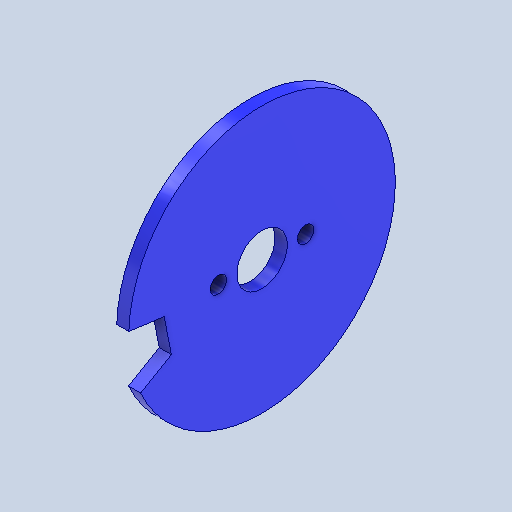
# Autodesk Inventor part: belt_liner_v1_3DP_P_F-1
Saved by Autodesk Inventor 2025.1 (Build 291241000, 241)
## iProperties
Created: 2024-12-16
Part Number: belt_liner_v1_3DP_P_F-1
Material: ABS プラスチック
Document SubType Name: Modeling
Designer: haruy
Density: 1.06 g/cm^3
Appearance: 青 - 壁塗料 - 光沢
Author: haruy
Autodesk Inventor part; units mm, degrees
ref_plane "YZ Plane" through (0, 0, 0) normal (1, 0, 0) x (0, 1, 0)
ref_plane "XZ Plane" through (0, 0, 0) normal (0, 1, 0) x (-1, 0, 0)
ref_plane "XY Plane" through (0, 0, 0) normal (0, 0, 1) x (1, 0, 0)
sketch "スケッチ1" plane through (0, 0, 0) normal (1, 0, 0) x (0, 1, 0)
  line L0 (-4.615, 22.6143) -> (-8.3061, 28.9627)
  arc A0 (-8.3061, 28.9627) -> (3.9037, 31.3913) centre (3.0245, 3.9054) ccw
  line L1 (3.9037, 31.3913) -> (2.923, 24.1137)
  line L2 (2.923, 24.1137) -> (-4.615, 22.6143)
  circle A1 centre (3.0245, -5.0946) radius 1.7
  circle A2 centre (3.0245, 12.9054) radius 1.7
  circle A3 centre (3.0245, 3.9054) radius 5.2
  point P0 (0, 0)
  constraints: 6 end point, 4 centre point, 2 point on circle
extrude "押し出し1" add sketch "スケッチ1" along normal blind 2.5
